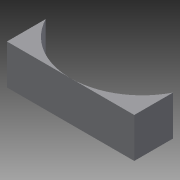
# Autodesk Inventor part: 知能ロボコン発射台つなぎ
Saved by Autodesk Inventor 2013 (Build 170138000, 138)
## iProperties
Created: 2014-05-30
Part Number: 知能ロボコン発射台つなぎ
Material: 一般
Document SubType Name: Modeling
Designer: horumo136
Density: 1 g/cm^3
Author: horumo136
Autodesk Inventor part; units mm, degrees
ref_plane "YZ Plane" through (0, 0, 0) normal (1, 0, 0) x (0, 1, 0)
ref_plane "XZ Plane" through (0, 0, 0) normal (0, 1, 0) x (-1, 0, 0)
ref_plane "XY Plane" through (0, 0, 0) normal (0, 0, 1) x (1, 0, 0)
sketch "スケッチ1" plane through (0, 0, 0) normal (0, 0, 1) x (1, 0, 0)
  line L0 (-5, 5) -> (-5, 29.3845)
  line L1 (-85, 5) -> (-85, 29.3845)
  arc A0 (-85, 29.3845) -> (-5, 29.3845) centre (-45, 50) ccw
  line L2 (-85, 5) -> (-5, 5)
  line L3 (-85, 5) -> (-5, 5)
  arc A1 (-85, 29.3845) -> (-5, 29.3845) centre (-45, 50) ccw
  line L4 (-85, 29.3845) -> (-85, 5)
  line L5 (-5, 29.3845) -> (-5, 5)
  line L6 (-5, 5) -> (-85, 5)
  line L7 (-85, 5) -> (-5, 5)
  line L8 (-5, 5) -> (-5, 29.3845)
  line L9 (-5, 29.3845) -> (-85, 29.3845)
  line L10 (-85, 29.3845) -> (-85, 5)
  arc A2 (-85, 29.3845) -> (-5, 29.3845) centre (-45, 50) ccw
  point P0 (0, 0)
  constraints: 22 end point, 6 point on circle, 5 equal length, 3 centre point, 1 concentric, 1 horizontal, 1 perpendicular
extrude "押し出し1" add sketch "スケッチ1" along normal blind 25 contours L2 A0 L0 | L2 L1 A0
